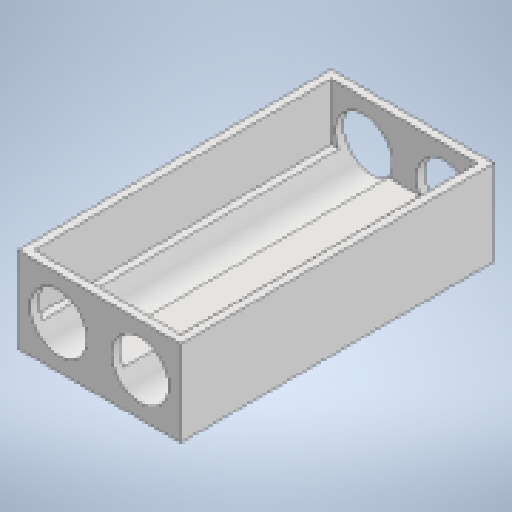
# Autodesk Inventor part: support pile
Saved by Autodesk Inventor 2024 (Build 280153000, 153)
## iProperties
Created: 2024-03-05
Part Number: support pile
Material: Générique
Document SubType Name: Modeling
Designer: phaly
Density: 1 g/cm^3
Appearance: Par défaut
Author: phaly
Autodesk Inventor part; units mm, degrees
ref_plane "YZ Plane" through (0, 0, 0) normal (1, 0, 0) x (0, 1, 0)
ref_plane "XZ Plane" through (0, 0, 0) normal (0, 1, 0) x (-1, 0, 0)
ref_plane "XY Plane" through (0, 0, 0) normal (0, 0, 1) x (1, 0, 0)
sketch "Esquisse1" plane through (0, 0, 0) normal (0, 0, 1) x (1, 0, 0)
  line L0 (0, 21) -> (41, 21)
  line L1 (41, 21) -> (41, 0)
  line L2 (41, 0) -> (0, 0)
  line L3 (0, 0) -> (0, 21)
  line L4 (-8.2, 0) -> (49.2, 0) projected
  line L5 (0, -4.2) -> (0, 25.2) projected
  point P0 (0, 0)
  dimension "d0" = 41
  dimension "d1" = 21
  constraints: 8 end point, 2 collinear, 2 parallel, 1 horizontal, 1 perpendicular
  measures "d0" distance of L0.start L0.end
  measures "d1" distance of L0.end L1.end
extrude "Extrusion1" add sketch "Esquisse1" along normal mid plane 77
sketch "Esquisse2" plane through (0, 0, 38.5) normal (0, 0, 1) x (1, 0, 0)
  circle A0 centre (10, 10.5) radius 7
  circle A1 centre (30, 10.5) radius 7
  line L0 (41, 21) -> (0, 21) projected
  line L1 (0, 21) -> (0, 0) projected
  line L2 (41, 0) -> (41, 21) projected
  line L3 (0, 0) -> (41, 0) projected
  dimension "d4" = 14
  dimension "d5" = 14
  dimension "d11" = 10.5
  dimension "d20" = 10.5
  dimension "d21" = 20
  constraints: 2 centre point
  measures "d4" diameter of A0
  measures "d5" diameter of A1
  measures "d11" distance from line of L3 A1.centre
  measures "d20" distance from line of L3 A0.centre
  measures "d21" distance of A1.centre A0.centre
extrude "Extrusion2" cut sketch "Esquisse2" against normal through all contours A0 | A1
sketch "Esquisse3" plane through (0, 21, 38.5) normal (0, 1, 0) x (1, 0, 0)
  line L0 (2, 75) -> (39, 75)
  line L1 (39, 75) -> (39, 2)
  line L2 (39, 2) -> (2, 2)
  line L3 (2, 2) -> (2, 75)
  line L4 (0, 77) -> (41, 77) projected
  line L5 (41, 0) -> (0, 0) projected
  line L6 (41, 77) -> (41, 0) projected
  line L7 (0, 77) -> (0, 0) projected
  point P0 (0, 38.5)
  dimension "d14" = 2
  dimension "d15" = 2
  dimension "d16" = 2
  dimension "d17" = 2
  constraints: 8 end point, 2 parallel, 1 horizontal, 1 perpendicular
  measures "d14" distance between parallel lines of L4 L0
  measures "d15" distance between parallel lines of L5 L2
  measures "d16" distance between parallel lines of L6 L1
  measures "d17" distance between parallel lines of L7 L3
extrude "Extrusion3" cut sketch "Esquisse3" against normal blind 14 contours L0 L1 L2 L3
sketch "Esquisse4" plane through (0, 7, 38.5) normal (0, 1, 0) x (1, 0, 0)
  line L0 (2, 75) -> (19, 75)
  line L1 (19, 75) -> (19, 2)
  line L2 (19, 2) -> (2, 2)
  line L3 (2, 2) -> (2, 75)
  line L4 (20.5, 75) -> (39, 75)
  line L5 (39, 75) -> (39, 2)
  line L6 (39, 2) -> (20.5, 2)
  line L7 (20.5, 2) -> (20.5, 75)
  line L8 (2, 75) -> (39, 75) projected
  line L9 (2, 2) -> (2, 75) projected
  line L10 (39, 75) -> (39, 2) projected
  line L11 (39, 2) -> (2, 2) projected
  point P0 (0, 38.5)
  dimension "d22" = 1.5
  dimension "d23" = 17
  constraints: 16 end point, 6 collinear, 4 parallel, 2 horizontal, 2 perpendicular
  measures "d22" distance between parallel lines of L7 L1
  measures "d23" distance of L1.end L2.end
extrude "Extrusion4" cut sketch "Esquisse4" against normal blind 5 contours L0 L1 L2 L3 | L4 L5 L6 L7
equation "\"d5\" = d4"
equation "\"d11\" = d20"
equation "\"d15\" = d14"
equation "\"d16\" = d15"
equation "\"d17\" = d16"
